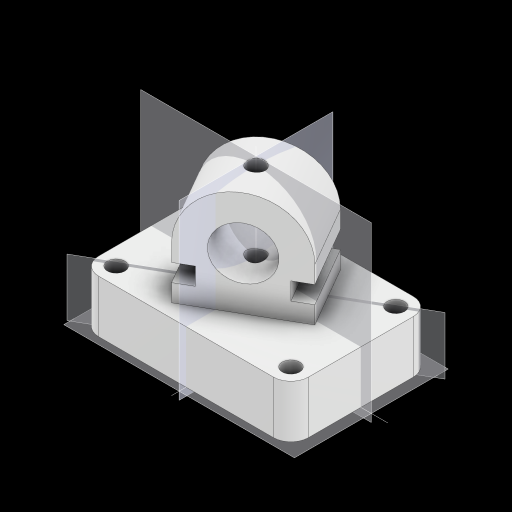
# Autodesk Inventor part: ANS9-TUT-BK
Saved by Autodesk Inventor 2024 (Build 280153000, 153)
## iProperties
Created: 2023-10-28
Part Number: ANS9-TUT-BK
Material: LCP Plastic
Document SubType Name: Modeling
Designer: bennk
Density: 1.626 g/cm^3
Appearance: Smooth - White
Mass: 151.354 g
Surface Area: 197.558 cm^2
Volume: 93.0834 cm^3
Author: bennk
Autodesk Inventor part; units mm, degrees
sketch "Sketch1" plane through (0, 0, 0) normal (0, 1, 0) x (-1, 0, 0)
  line L0 (31.75, -25.4) -> (-31.75, -25.4)
  line L1 (-38.1, -19.05) -> (-38.1, 19.05)
  line L2 (-31.75, 25.4) -> (31.75, 25.4)
  line L3 (38.1, 19.05) -> (38.1, -19.05)
  arc A0 (38.1, 19.05) -> (31.75, 25.4) centre (31.75, 19.05) ccw
  arc A1 (31.75, -25.4) -> (38.1, -19.05) centre (31.75, -19.05) ccw
  arc A2 (-38.1, -19.05) -> (-31.75, -25.4) centre (-31.75, -19.05) ccw
  arc A3 (-31.75, 25.4) -> (-38.1, 19.05) centre (-31.75, 19.05) ccw
  circle A4 centre (31.75, -19.05) radius 3.175
  circle A5 centre (-31.75, -19.05) radius 3.175
  circle A6 centre (-31.75, 19.05) radius 3.175
  circle A7 centre (31.75, 19.05) radius 3.175
  line L4 (0, 25.4) -> (0, -25.4) construction
  line L5 (38.1, 0) -> (-38.1, 0) construction
  point P0 (0, 0)
  point P1 (0, 0)
  dimension "d0" = 6.35
  dimension "d1" = 6.35
  dimension "d2" = 76.2
  dimension "d3" = 50.8
  dimension "d4" = 38.1
  dimension "d5" = 25.4
  constraints: 12 end point, 8 centre point, 8 point on circle, 8 tangent, 6 equal radius, 6 midpoint, 4 coincident, 2 parallel, 1 horizontal, 1 perpendicular
  measures "d0" radius of A0
  measures "d1" diameter of A4
  measures "d2" distance between parallel lines of L1 L3
  measures "d3" distance between parallel lines of L0 L2
  measures "d4" distance from line of point (0, 0) L3
  measures "d5" distance from line of point (0, 0) L2
extrude "MAIN BODY" add sketch "Sketch1" along normal blind 19.05
ref_plane "WP1" through (0, 0, 0) normal (0.5, 0, 0.866) x (0, 1, 0)
sketch "Sketch2" plane through (0, 0, 0) normal (0.5, 0, 0.866) x (0, 1, 0)
  line L0 (19.05, -40.1963) -> (19.05, 14.7963) construction
  line L1 (19.05, 19.05) -> (25.4, 19.05)
  line L2 (25.4, 19.05) -> (25.4, 12.7)
  line L3 (25.4, 12.7) -> (31.75, 12.7)
  line L4 (31.75, 12.7) -> (31.75, 19.05)
  line L5 (31.75, 19.05) -> (38.1, 19.05)
  line L6 (38.1, 19.05) -> (38.1, -19.05)
  line L7 (38.1, -19.05) -> (31.75, -19.05)
  line L8 (31.75, -19.05) -> (31.75, -12.7)
  line L9 (31.75, -12.7) -> (25.4, -12.7)
  line L10 (25.4, -12.7) -> (25.4, -19.05)
  line L11 (25.4, -19.05) -> (19.05, -19.05)
  line L12 (19.05, -19.05) -> (19.05, 19.05)
  arc A0 (38.1, -19.05) -> (38.1, 19.05) centre (38.1, 0) ccw
  circle A1 centre (38.1, 0) radius 9.525
  point P0 (0, 0)
  dimension "d9" = 19.05
  dimension "d10" = 6.35
  dimension "d11" = 6.35
  dimension "d13" = 6.35
  dimension "d14" = 6.35
  dimension "d15" = 38.1
  dimension "d17" = 19.05
  dimension "d18" = 6.35
  dimension "d19" = 6.35
  dimension "d20" = 19.05
  constraints: 24 end point, 9 perpendicular, 7 point on line, 2 centre point, 2 horizontal, 2 point on circle, 1 coincident, 1 collinear, 1 tangent
  measures "d9" distance between parallel lines of L0 L6
  measures "d10" distance between parallel lines of L10 L8
  measures "d11" distance of L6.end L7.end
  measures "d13" distance of L2.end L3.end
  measures "d14" distance between parallel lines of L6 L4
  measures "d15" distance of L5.end L6.end
  measures "d17" distance from line of point (0, 0) L11
  measures "d18" distance between parallel lines of L11 L9
  measures "d19" distance between parallel lines of L5 L3
  measures "d20" diameter of A1
extrude "TOP BOSS" add sketch "Sketch2" along normal mid plane 25.4 contours L1 L2 L3 L4 L5 L6 A1 L7 L8 L9 L10 L11 L12 | A0 L6 A1
sketch "Sketch6" plane through (0, 0, 0) normal (0, -1, 0) x (1, 0, 0)
  point P0 (0, 0)
  point P1 (0, 0)
  constraints: 1 coincident
hole "THROUGH HOLE" at (0, 0, 0) direction (0, 1, 0) diameter 6.35 end through all
equation "\"d11\" = d10"
equation "\"d13\" = d10"
equation "\"d14\" = d11"
equation "\"d17\" = 0.5 * d15"
equation "\"d18\" = d10"
equation "\"d19\" = d18"
body "Solid1"
